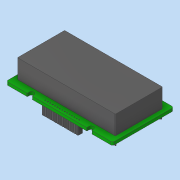
# Autodesk Inventor part: Display
Saved by Autodesk Inventor 2018 (Build 220112000, 112)
## iProperties
Created: 2020-10-03
Part Number: Display
Material: Generisch
Document SubType Name: Modeling
Designer: marce
Density: 1 g/cm^3
Appearance: Siliziumnitrid - poliert
Author: marce
Autodesk Inventor part; units mm, degrees
ref_plane "YZ Plane" through (0, 0, 0) normal (1, 0, 0) x (0, 1, 0)
ref_plane "XZ Plane" through (0, 0, 0) normal (0, 1, 0) x (-1, 0, 0)
ref_plane "XY Plane" through (0, 0, 0) normal (0, 0, 1) x (1, 0, 0)
sketch "Skizze1" plane through (0, 0, 0) normal (0, 0, 1) x (1, 0, 0)
  line L0 (0, 0) -> (55.7, 0)
  line L1 (55.7, 0) -> (55.7, 32)
  line L2 (55.7, 32) -> (0, 32)
  line L3 (0, 32) -> (0, 0)
  dimension "d0" = 55.7
  dimension "d1" = 32
  constraints: 8 end point, 2 parallel, 1 horizontal, 1 perpendicular
  measures "d0" distance of L2.end L1.end
  measures "d1" distance of L1.end L0.end
extrude "Extrusion1" add sketch "Skizze1" along normal blind 1.6
sketch "Skizze2" plane through (0, 0, 1.6) normal (0, 0, 1) x (1, 0, 0)
  line L0 (11, 0) -> (13.5, 0)
  line L1 (13.5, 0) -> (13.5, 1)
  line L2 (13.5, 1) -> (11, 1)
  line L3 (11, 1) -> (11, 0)
  arc A0 (13.5, 1) -> (11, 1) centre (12.25, 1) ccw
  line L4 (0, 32) -> (0, 0) projected
  line L5 (0, 0) -> (55.7, 0) projected
  line L6 (42.2, 0) -> (44.7, 0)
  line L7 (44.7, 0) -> (44.7, 1)
  line L8 (44.7, 1) -> (42.2, 1)
  line L9 (42.2, 1) -> (42.2, 0)
  arc A1 (44.7, 1) -> (42.2, 1) centre (43.45, 1) ccw
  line L10 (55.7, 32) -> (0, 32) projected
  line L11 (11, 32) -> (13.5, 32)
  line L12 (13.5, 32) -> (13.5, 31)
  line L13 (13.5, 31) -> (11, 31)
  line L14 (11, 31) -> (11, 32)
  arc A2 (11, 31) -> (13.5, 31) centre (12.25, 31) ccw
  line L15 (42.2, 32) -> (44.7, 32)
  line L16 (44.7, 32) -> (44.7, 31)
  line L17 (44.7, 31) -> (42.2, 31)
  line L18 (42.2, 31) -> (42.2, 32)
  arc A3 (42.2, 31) -> (44.7, 31) centre (43.45, 31) ccw
  dimension "d8" = 2.5
  dimension "d9" = 12.25
  dimension "d10" = 1.25
  dimension "d11" = 1
  dimension "d12" = 2.5
  dimension "d13" = 1.25
  dimension "d14" = 1
  dimension "d15" = 31.2
  dimension "d19" = 2.5
  dimension "d20" = 1
  dimension "d21" = 12.25
  dimension "d22" = 2.5
  dimension "d23" = 1
  dimension "d24" = 31.2
  constraints: 32 end point, 8 parallel, 8 point on circle, 4 centre point, 4 horizontal, 4 midpoint, 4 perpendicular, 3 collinear, 1 point on line
  measures "d8" distance of L2.end L1.end
  measures "d9" distance from line of L4 A0.centre
  measures "d10" radius of A0
  measures "d11" distance of L2.end L0.start
  measures "d12" distance of L8.end L7.end
  measures "d13" radius of A1
  measures "d14" distance of L8.end L6.start
  measures "d15" distance between parallel lines of L3 L9
  measures "d19" distance of L12.end L13.end
  measures "d20" distance of L11.end L12.end
  measures "d21" distance from line of L4 A2.centre
  measures "d22" distance of L16.end L17.end
  measures "d23" distance of L16.start L16.end
  measures "d24" distance between parallel lines of L18 L14
extrude "Extrusion2" cut sketch "Skizze2" against normal through all
sketch "Skizze3" plane through (0, 0, 1.6) normal (0, 0, 1) x (1, 0, 0)
  line L0 (0, 0) -> (18.96, 0)
  line L1 (18.96, 0) -> (18.96, 1.5)
  line L2 (18.96, 1.5) -> (0, 1.5)
  line L3 (0, 1.5) -> (0, 0)
  dimension "d27" = 18.96
  dimension "d28" = 1.5
  constraints: 8 end point, 2 parallel, 1 horizontal, 1 perpendicular
  measures "d27" distance of L2.end L1.end
  measures "d28" distance of L1.end L0.end
hole "Bohrung1" at (18.96, 1.5, 1.6) direction (0, 0, -1) diameter 0.5 end through all
pattern_linear "Rechteckige Anordnung1" count 15 spacing 1.27 along (1, 0, 0) of "Bohrung1"
sketch "Skizze4" plane through (0, 0, 1.6) normal (0, 0, 1) x (1, 0, 0)
  line L0 (2.2, 28.35) -> (53.5, 28.35)
  line L1 (53.5, 28.35) -> (53.5, 3.65)
  line L2 (53.5, 3.65) -> (2.2, 3.65)
  line L3 (2.2, 3.65) -> (2.2, 28.35)
  line L4 (0, 32) -> (0, 0) projected
  line L5 (42.2, 32) -> (13.5, 32) projected
  point P0 (2.2, 16)
  point P1 (0, 16)
  point P2 (27.85, 28.35)
  point P3 (27.85, 32)
  dimension "d41" = 51.3
  dimension "d42" = 24.7
  constraints: 8 end point, 4 midpoint, 2 parallel, 1 horizontal, 1 horizontal alignment, 1 perpendicular, 1 vertical alignment
  measures "d41" distance of L1.end L2.end
  measures "d42" distance of L0.end L1.end
extrude "Extrusion3" add sketch "Skizze4" along normal blind 9.9
sketch "Skizze5" plane through (0, 0, 0) normal (0, 0, -1) x (-1, 0, 0)
  line L0 (-53.5, 28.35) -> (-2.2, 28.35) projected
  line L1 (-2.2, 28.35) -> (-2.2, 3.65) projected
  line L2 (-2.2, 3.65) -> (-53.5, 3.65) projected
  line L3 (-53.5, 3.65) -> (-53.5, 28.35) projected
  line L4 (-53.1464, 28.35) -> (-53.5, 27.9964)
  line L5 (-53.5, 27.9964) -> (-49.2574, 23.7538)
  line L6 (-49.2574, 23.7538) -> (-48.9038, 24.1074)
  line L7 (-48.9038, 24.1074) -> (-53.1464, 28.35)
  line L8 (-53.5, 3.65) -> (-53.5, 28.35) projected
  line L9 (-53.5, 4.0036) -> (-53.1464, 3.65)
  line L10 (-53.1464, 3.65) -> (-48.9038, 7.8926)
  line L11 (-48.9038, 7.8926) -> (-49.2574, 8.2462)
  line L12 (-49.2574, 8.2462) -> (-53.5, 4.0036)
  line L13 (-2.2, 4.0036) -> (-2.5536, 3.65)
  line L14 (-2.5536, 3.65) -> (-6.7962, 7.8926)
  line L15 (-6.7962, 7.8926) -> (-6.4426, 8.2462)
  line L16 (-6.4426, 8.2462) -> (-2.2, 4.0036)
  line L17 (-2.2, 3.65) -> (-2.2, 28.35) projected
  line L18 (-2.5536, 28.35) -> (-2.2, 27.9964)
  line L19 (-2.2, 27.9964) -> (-6.4426, 23.7538)
  line L20 (-6.4426, 23.7538) -> (-6.7962, 24.1074)
  line L21 (-6.7962, 24.1074) -> (-2.5536, 28.35)
  line L22 (-27.2536, 28.35) -> (-26.7536, 28.35)
  line L23 (-26.7536, 28.35) -> (-26.7536, 22.35)
  line L24 (-26.7536, 22.35) -> (-27.2536, 22.35)
  line L25 (-27.2536, 22.35) -> (-27.2536, 28.35)
  line L26 (-28.1, 3.65) -> (-27.6, 3.65)
  line L27 (-27.6, 3.65) -> (-27.6, 9.65)
  line L28 (-27.6, 9.65) -> (-28.1, 9.65)
  line L29 (-28.1, 9.65) -> (-28.1, 3.65)
  line L30 (-53.5, 28.35) -> (-53.5, 3.65) projected
  point P0 (0, 0)
  point P1 (-27.85, 3.65)
  dimension "d45" = 6
  dimension "d46" = 0.5
  dimension "d47" = 45
  dimension "d48" = 0.3535
  dimension "d49" = 0.3535
  dimension "d50" = 6
  dimension "d51" = 45
  dimension "d52" = 45
  constraints: 48 end point, 13 parallel, 13 point on line, 9 equal length, 6 perpendicular, 2 midpoint
  measures "d45" distance of L6.end L4.start
  measures "d46" distance of L5.end L6.end
  measures "d47" angle of L0 L7
  measures "d48" distance of L4.start L0.start
  measures "d49" distance of L4.end L0.start
  measures "d50" distance of L22.end L23.end
  measures "d51" angle of L2 L10
  measures "d52" angle of L14 L2
extrude "Extrusion4" add sketch "Skizze5" along normal blind 3 contours L7 L6 L5 L4 | L0 L23 L24 L25 | L12 L11 L10 L9 | L18 L19 L20 L21 | L29 L28 L27 L2 | L13 L14 L15 L16
sketch "Skizze6" plane through (0, 0, 0) normal (0, 0, -1) x (-1, 0, 0)
  circle A0 centre (-18.96, 1.5) radius 0.25 projected
  line L0 (-18.96, 1.5) -> (-18.96, 0.23)
  line L1 (-18.96, 2.77) -> (-18.325, 2.77)
  line L2 (-18.325, 2.77) -> (-18.325, 0.23)
  line L3 (-18.325, 0.23) -> (-18.96, 0.23)
  line L4 (-18.96, 0.23) -> (-19.595, 0.23)
  line L5 (-19.595, 0.23) -> (-19.595, 2.77)
  line L6 (-19.595, 2.77) -> (-18.96, 2.77)
  line L7 (-18.325, 0.48) -> (-18.575, 0.23)
  line L8 (-18.325, 2.52) -> (-18.575, 2.77)
  line L9 (-19.345, 2.77) -> (-19.595, 2.52)
  line L10 (-19.345, 0.23) -> (-19.595, 0.48)
  point P0 (0, 0)
  dimension "d57" = 1.27
  dimension "d58" = 1.27
  dimension "d59" = 0.635
  dimension "d60" = 2.54
  dimension "d61" = 90
  dimension "d62" = 0.635
  dimension "d63" = 2.54
  dimension "d64" = 0.635
  dimension "d65" = 45
  dimension "d66" = 0.25
  dimension "d67" = 45
  dimension "d68" = 0.25
  dimension "d69" = 0.25
  dimension "d70" = 45
  dimension "d71" = 45
  dimension "d72" = 0.25
  constraints: 22 end point, 10 point on line, 2 perpendicular, 1 collinear, 1 vertical
  measures "d57" distance of L0.start L0.end
  measures "d58" distance of L0.start L1.start
  measures "d59" distance of L1.start L1.end
  measures "d60" distance of L1.end L2.end
  measures "d61" angle of L1 L2
  measures "d62" distance of L0.end L4.end
  measures "d63" distance of L4.end L5.end
  measures "d64" distance from line of L2 L0.start
  measures "d65" angle of L3 L7
  measures "d66" distance from line of L7.end L2
  measures "d67" angle of L1 L8
  measures "d68" distance from line of L2 L8.end
  measures "d69" horizontal distance of L9.start L9.end
  measures "d70" angle of L5 L9
  measures "d71" angle of L4 L10
  measures "d72" distance from line of L5 L10.start
extrude "Extrusion5" add sketch "Skizze6" along normal blind 4.57 contours L4 L10 L5 L9 L6 L1 L8 L2 L7 L3
pattern_linear "Rechteckige Anordnung2" count 15 spacing 1.27 along (1, 0, 0) of "Extrusion5"
fillet "Rundung1" radius 1 4 edges at (0, 0, 0.8) (0, 32, 0.8) (55.7, 0, 0.8) (55.7, 32, 0.8)
fillet "Rundung1" radius 0.2 12 edges at (42.2, 32, 0.8) (44.7, 32, 0.8) (11, 32, 0.8) (13.5, 32, 0.8) (13.5, 0, 0.8) (11, 0, 0.8) (42.2, 0, 0.8) (44.7, 0, 0.8) (2.2, 3.65, 6.55) (53.5, 3.65, 6.55) (53.5, 28.35, 6.55) (2.2, 28.35, 6.55)
